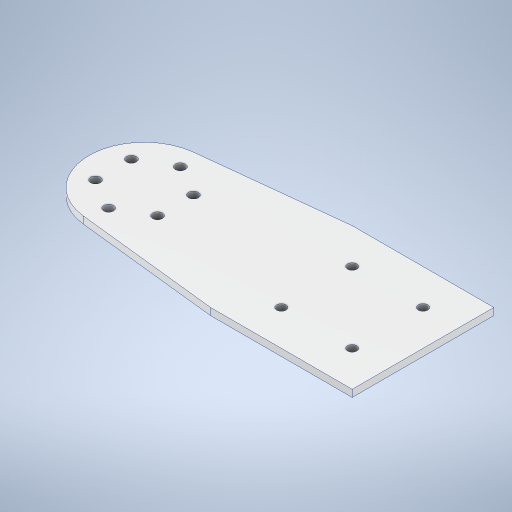
# Autodesk Inventor part: link3_plate1
Saved by Autodesk Inventor 2024 (Build 280153000, 153)
## iProperties
Created: 2024-12-13
Part Number: link3_plate1
Material: アルミニウム 6061
Document SubType Name: Modeling
Designer: hirek
Density: 2.7 g/cm^3
Appearance: アルミニウム - フラット
Author: hirek
Autodesk Inventor part; units mm, degrees
ref_plane "YZ Plane" through (0, 0, 0) normal (1, 0, 0) x (0, 1, 0)
ref_plane "XZ Plane" through (0, 0, 0) normal (0, 1, 0) x (-1, 0, 0)
ref_plane "XY Plane" through (0, 0, 0) normal (0, 0, 1) x (1, 0, 0)
sketch "スケッチ1" plane through (0, 0, 0) normal (0, 1, 0) x (-1, 0, 0)
  line L0 (0, 0) -> (65.5, 0)
  line L1 (65.5, 0) -> (65.5, -70)
  line L2 (65.5, -70) -> (0, -70)
  line L3 (0, -70) -> (0, 0)
  dimension "d0" = 65.5
  dimension "d1" = 70
  constraints: 8 end point, 2 parallel, 1 horizontal, 1 perpendicular
  measures "d0" distance of L1.end L2.end
  measures "d1" distance of L0.end L1.end
extrude "押し出し1" add sketch "スケッチ1" along normal blind 3
sketch "スケッチ3" plane through (0, 3, 0) normal (0, 1, 0) x (1, 0, 0)
  line L0 (-65.5, 0) -> (0, 0) projected
  line L1 (-32.75, 0) -> (-32.75, 70)
  line L2 (0, 70) -> (-65.5, 70) projected
  circle A0 centre (-32.75, 35) radius 15.18
  point P0 (-32.75, 50.18)
  point P1 (-45.8963, 42.59)
  point P2 (-45.8963, 27.41)
  point P3 (-32.75, 19.82)
  point P4 (-19.6037, 27.41)
  point P5 (-19.6037, 42.59)
  dimension "d15" = 30.36
  dimension "d18" = 360
  constraints: 3 midpoint, 2 end point, 1 point on line, 1 vertical alignment, 9 other
hole "穴2" at (-32.75, 3, -50.18) at (-45.8963, 3, -42.59) at (-45.8963, 3, -27.41) at (-32.75, 3, -19.82) at (-19.6037, 3, -27.41) at (-19.6037, 3, -42.59) direction (0, -1, 0) diameter 4.2 end through all
sketch "スケッチ4" plane through (0, 3, 0) normal (0, 1, 0) x (1, 0, 0)
  line L0 (-65.5, 70) -> (-65.5, 0) projected
  line L1 (0, 70) -> (-65.5, 70) projected
  circle A0 centre (-32.75, 35) radius 23.5
  line L2 (0, 0) -> (0, 70) projected
  line L3 (-65.5, 70) -> (0, 70)
  line L4 (0, 70) -> (0, 0)
  line L5 (0, 0) -> (-65.5, 0)
  line L6 (-65.5, 0) -> (-65.5, 70)
  dimension "d27" = 47
  dimension "d28" = 35
  dimension "d29" = 32.75
  constraints: 8 end point, 2 parallel, 1 centre point, 1 horizontal, 1 perpendicular
  measures "d27" diameter of A0
  measures "d28" distance from line of A0.centre L1
  measures "d29" distance from line of L2 A0.centre
extrude "押し出し2" cut sketch "スケッチ4" against normal blind 3
sketch "スケッチ5" plane through (-32.75, 3, -35) normal (0, 1, 0) x (1, 0, 0)
  line L0 (58, 30) -> (118, 30)
  line L1 (118, 30) -> (118, -30)
  line L2 (118, -30) -> (58, -30)
  line L3 (58, -30) -> (58, 30)
  circle A0 centre (0, 0) radius 23.5 projected
  line L4 (58, 30) -> (-2.5612, 23.36)
  circle A1 centre (0, 0) radius 23.5
  line L5 (58, -30) -> (-2.5612, -23.36)
  point P0 (32.75, -35)
  point P1 (-2.5612, -23.36)
  dimension "d32" = 60
  dimension "d33" = 60
  dimension "d34" = 30
  dimension "d35" = 58
  constraints: 12 end point, 2 coincident, 2 parallel, 1 horizontal, 1 perpendicular, 7 other
  measures "d32" distance of L1.end L2.end
  measures "d33" distance of L0.end L1.end
  measures "d34" distance from line of L0 point (0, 0)
  measures "d35" distance from line of L3 point (0, 0)
extrude "押し出し3" add sketch "スケッチ5" against normal blind 3 contours L0 L1 L2 L3 | L3 L5 A0 L4
sketch "スケッチ6" plane through (0, 3, 0) normal (0, 1, 0) x (1, 0, 0)
  line L0 (40.25, 50) -> (70.25, 50)
  line L1 (70.25, 50) -> (70.25, 20)
  line L2 (70.25, 20) -> (40.25, 20)
  line L3 (40.25, 20) -> (40.25, 50)
  line L4 (85.25, 65) -> (25.25, 65) projected
  point P0 (0, 0)
  dimension "d38" = 30
  dimension "d39" = 30
  dimension "d40" = 15
  dimension "d41" = 15
  constraints: 8 end point, 4 coincident, 2 parallel, 1 horizontal, 1 perpendicular
  measures "d38" distance of L1.end L2.end
  measures "d39" distance of L0.end L1.end
  measures "d40" distance between parallel lines of L0 L4
  measures "d41" distance from line of L3 L4.end
hole "穴3" at (70.25, 3, -50) at (40.25, 3, -50) at (40.25, 3, -20) at (70.25, 3, -20) direction (0, -1, 0) diameter 4 end through all
